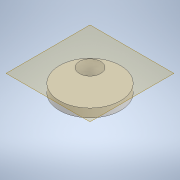
# Autodesk Inventor part: adaptator_potentiometre_test_1
Saved by Autodesk Inventor 2020.1 (Build 241239000, 239)
## iProperties
Created: 2019-07-23
Part Number: adaptator_potentiometre_test_1
Material: Générique
Document SubType Name: Modeling
Designer: marlo
Density: 1 g/cm^3
Appearance: Par défaut
Author: marlo
Autodesk Inventor part; units mm, degrees
ref_plane "YZ Plane" through (0, 0, 0) normal (1, 0, 0) x (0, 1, 0)
ref_plane "XZ Plane" through (0, 0, 0) normal (0, 1, 0) x (-1, 0, 0)
ref_plane "XY Plane" through (0, 0, 0) normal (0, 0, 1) x (1, 0, 0)
sketch "Esquisse1" plane through (0, 0, 0) normal (0, 1, 0) x (-1, 0, 0)
  circle A0 centre (0, 0) radius 18
  dimension "d0" = 36
  constraints: 1 centre point
  measures "d0" diameter of A0
extrude "Extrusion1" add sketch "Esquisse1" along normal blind 5
sketch "Esquisse3" plane through (0, 0, 0) normal (0, -1, 0) x (1, 0, 0)
  line L0 (-3.5, 0.5) -> (3.5, 0.5)
  line L1 (3.5, 0.5) -> (3.5, -0.5)
  line L2 (3.5, -0.5) -> (-3.5, -0.5)
  line L3 (-3.5, -0.5) -> (-3.5, 0.5)
  line L4 (-3.5, 0.5) -> (3.5, -0.5) construction
  line L5 (3.5, 0.5) -> (-3.5, -0.5) construction
  circle A0 centre (0, 0) radius 3.5
  circle A1 centre (0, 0) radius 7.5
  point P0 (3.4641, 0.5)
  point P1 (-3.4641, 0.5)
  point P2 (3.4641, -0.5)
  point P3 (-3.4641, -0.5)
  dimension "d12" = 1
  dimension "d14" = 7
  dimension "d15" = 4
  constraints: 12 end point, 2 centre point, 2 coincident, 2 midpoint, 2 parallel, 1 horizontal, 1 perpendicular, 1 tangent
  measures "d12" distance of L0.end L1.end
  measures "d14" diameter of A0
  measures "d15" radial gap between concentric circles of A1 A0
extrude "Extrusion2" add sketch "Esquisse3" along normal blind 7 contours L0 A0 L3 | L0 A0 L2 | A0 L2 L3 | L0 L1 A0 | L1 L2 A0 | A1
ref_plane "Plan de construction1" through (0, 10, 0) normal (0, 1, 0) x (1, 0, 0)
sketch "Esquisse4" plane through (0, 10, 0) normal (0, 1, 0) x (1, 0, 0)
  line L0 (0, 0) -> (0, 22.3046) construction
  line L1 (-26.1226, 0) -> (0, 0) construction
  line L2 (-3.4641, 0.5) -> (3.4641, 0.5) projected
  arc A0 (0, 8) -> (-16, 8) centre (-8, 8) ccw
  line L3 (-16, 8) -> (0, 8)
  line L4 (-37.5536, 8) -> (28.7867, 8)
  dimension "d19" = 8
  dimension "d20" = 8
  dimension "d21" = 8
  constraints: 8 end point, 2 collinear, 2 parallel, 2 point on circle, 1 centre point, 1 midpoint, 1 vertical
  measures "d19" distance from line of A0.centre L0
  measures "d20" distance from line of L1 A0.centre
  measures "d21" distance of A0.centre L3.end
revolve "Révolution2" cut sketch "Esquisse4" angle 360 about axis through (-37.5536, 10, -8) along (1, 0, 0)
